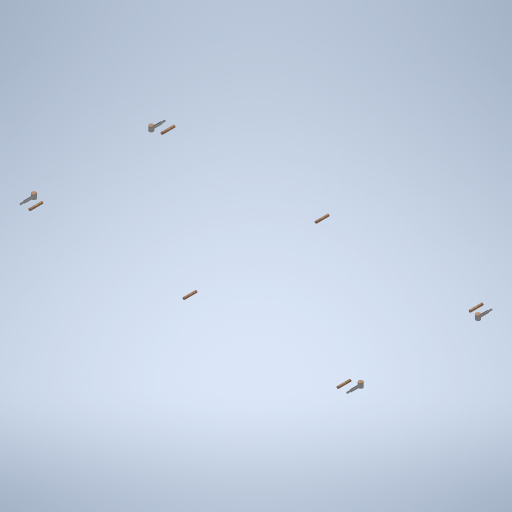
# Autodesk Inventor part: Minifixes pull Side Boards-04
Saved by Autodesk Inventor 2024.3 (Build 283343000, 343)
## iProperties
RuleStatus: InUse
Created: 2014-05-08
Part Number: Minifixes pull Side Boards-04
Material: Generic
Document SubType Name: Modeling
Designer: SauliusD
Density: 1 g/cm^3
Appearance: Default
AfterDocNew0: Fire Form
Author: SauliusD
Autodesk Inventor part; units mm, degrees
sketch "Sketch2" plane through (0, 0, 0) normal (0, 0, 1) x (1, 0, 0)
  line L0 (-178.2411, -363.1253) -> (-1324.2411, -363.1253)
  line L1 (-1324.2411, -363.1253) -> (-1324.2411, 106.8747)
  line L2 (-1324.2411, 106.8747) -> (-178.2411, 106.8747)
  line L3 (-178.2411, 106.8747) -> (-178.2411, -363.1253)
  point P0 (-751.2411, 106.8747)
  point P1 (-1324.2411, -128.1253)
  constraints: 8 end point, 2 midpoint, 2 parallel, 1 horizontal, 1 perpendicular
ref_plane "Work Plane1" through (0, 0, -9) normal (0, 0, 1) x (1, 0, 0)
sketch "Sketch3" plane through (0, 0, -9) normal (0, 0, 1) x (1, 0, 0)
  line L0 (-178.2411, 106.8747) -> (-178.2411, -363.1253) construction
  line L1 (-1324.2411, 106.8747) -> (-178.2411, 106.8747) construction
  line L2 (-1324.2411, -363.1253) -> (-1324.2411, 106.8747) construction
  line L3 (-1311.2411, 106.8747) -> (-1307.2411, 106.8747)
  line L4 (-1307.2411, 106.8747) -> (-1307.2411, 72.8747)
  line L5 (-1307.2411, 72.8747) -> (-1311.2411, 72.8747)
  line L6 (-1311.2411, 72.8747) -> (-1311.2411, 106.8747)
  line L7 (-1311.2411, 106.8747) -> (-1308.7411, 106.8747)
  line L8 (-1308.7411, 106.8747) -> (-1308.7411, 119.8747)
  line L9 (-1308.7411, 119.8747) -> (-1311.2411, 119.8747)
  line L10 (-1311.2411, 119.8747) -> (-1311.2411, 106.8747)
  line L11 (-751.2411, 106.8747) -> (-751.2411, 132.7708) construction
  line L12 (-191.2411, 72.8747) -> (-191.2411, 106.8747)
  point P0 (0, 0)
  dimension "d5" = 8
  dimension "d7" = 5
  dimension "d8" = 13
  dimension "Dist_Between_Planes" = 1146
  dimension "Distance_between_Axis" = 1120
  constraints: 20 end point, 5 parallel, 2 horizontal, 2 perpendicular, 2 symmetric about line, 1 collinear, 1 midpoint, 1 vertical alignment
  measures "d5" diameter of L4 L6
  measures "d7" diameter of L8 L10
  measures "d8" distance of L7.end L8.end
  measures "Dist_Between_Planes" distance of L1.start L0.start
  measures "Distance_between_Axis" distance between parallel lines of L6 L12
revolve "Minifix Revolve" add sketch "Sketch3" angle 360 about axis through (-1311.2411, 119.8747, -9) along (0, -1, 0)
sketch "Sketch4" plane through (0, 0, -9) normal (0, 0, 1) x (1, 0, 0)
  line L0 (-1315.2411, 72.8747) -> (-1307.2411, 72.8747) construction
  circle A0 centre (-1311.2411, 72.8747) radius 7.5
  point P0 (0, 0)
  dimension "d10" = 15
  constraints: 1 centre point, 1 midpoint
  measures "d10" diameter of A0
extrude "Minifix Extrude" add sketch "Sketch4" along normal up to surface (9 mm away)
extrude "Minifix extrude 2" add sketch "Sketch4" against normal blind 6
ref_plane "Work Plane2" through (-751.2411, 106.8747, 0) normal (1, 0, 0) x (0, 1, 0)
ref_plane "Work Plane3" through (-1324.2411, -128.1253, 0) normal (0, 1, 0) x (-1, 0, 0)
sketch "Sketch5" plane through (0, 0, -9) normal (0, 0, 1) x (1, 0, 0)
  line L0 (-1311.2411, 216.4747) -> (-1311.2411, -459.7253) construction
  line L1 (-1279.2411, 119.8747) -> (-1279.2411, 76.8747)
  line L2 (-1279.2411, 119.8747) -> (-1275.2411, 119.8747)
  line L3 (-1275.2411, 119.8747) -> (-1275.2411, 76.8747)
  line L4 (-1275.2411, 76.8747) -> (-1279.2411, 76.8747)
  line L5 (-1313.7411, 119.8747) -> (-1308.7411, 119.8747) construction
  line L6 (-1315.2411, 106.8747) -> (-1307.2411, 106.8747) construction
  point P0 (0, 0)
  dimension "Dowel_D" = 8
  dimension "Dowel_Drill_Depth" = 30
  dimension "d17" = 32
  constraints: 8 end point, 2 parallel, 2 perpendicular, 1 collinear
  measures "Dowel_D" diameter of L3 L1
  measures "Dowel_Drill_Depth" distance between parallel lines of L4 L6
  measures "d17" distance from line of L1.start L0
revolve "Dowel Revolve" add sketch "Sketch5" angle 360 about axis through (-1279.2411, 119.8747, -9) along (0, -1, 0) separate body
mirror "Mirror1" about plane through (-751.2411, 106.8747, 0) normal (1, 0, 0) of "Minifix Extrude", "Minifix Revolve", "Dowel Revolve", "Minifix extrude 2" bodies 1
sketch "Sketch6" plane through (0, 0, -9) normal (0, 0, 1) x (1, 0, 0)
  point P0 (0, 0)
sketch "Sketch7" plane through (0, 0, -9) normal (0, 0, 1) x (1, 0, 0)
  line L0 (-751.2411, 216.4747) -> (-751.2411, -459.7253) construction
  line L1 (-751.2411, 119.8747) -> (-747.2411, 119.8747)
  line L2 (-747.2411, 119.8747) -> (-747.2411, 76.8747)
  line L3 (-747.2411, 76.8747) -> (-751.2411, 76.8747)
  line L4 (-751.2411, 76.8747) -> (-751.2411, 119.8747)
  line L5 (-1313.7411, 119.8747) -> (-1308.7411, 119.8747) construction
  line L6 (-1315.2411, 106.8747) -> (-1307.2411, 106.8747) construction
  line L7 (-1283.2411, 76.8747) -> (-1275.2411, 76.8747) projected
  line L8 (-1283.2411, 119.8747) -> (-1275.2411, 119.8747) projected
  point P0 (0, 0)
  point P1 (-751.2411, -459.7253)
  dimension "d46" = 8
  constraints: 8 end point, 2 collinear, 2 parallel, 1 horizontal, 1 perpendicular, 1 vertical, 1 other
  measures "d46" diameter of L2 L4
revolve "Center Dowel Revolve" add sketch "Sketch7" angle 360 about axis through (-751.2411, 106.8747, -9) along (0, -1, 0) separate body
ref_plane "Work Plane4" through (-178.2411, 106.8747, 0) normal (0, 1, 0) x (-1, 0, 0)
mirror "Mirror2" about plane through (-1324.2411, -128.1253, 0) normal (0, 1, 0) of "Minifix Extrude", "Minifix Revolve", "Dowel Revolve", "Minifix extrude 2", "Mirror1" bodies 1
mirror "Mirror Center" about plane through (-1324.2411, -128.1253, 0) normal (0, 1, 0) of "Center Dowel Revolve" bodies 3
sketch "Sketch9" plane through (-1311.2411, 72.8747, 0) normal (0, 0, 1) x (1, 0, 0)
  circle A0 centre (0, 0) radius 7.5 projected
  point P0 (1311.2411, -72.8747)
extrude "Side Cover Cap Extrusion" add sketch "Sketch9" along normal blind 2 separate body
fillet "Side Cover Cap Fillet" radius 1.6 1 edges at (-1318.7411, 72.8747, 2)
mirror "Mirror3" about plane through (-751.2411, 106.8747, 0) normal (1, 0, 0) of "Side Cover Cap Extrusion", "Side Cover Cap Fillet" bodies 4
mirror "Mirror4" about plane through (-1324.2411, -128.1253, 0) normal (0, 1, 0) of "Side Cover Cap Extrusion", "Side Cover Cap Fillet", "Mirror3" bodies 4
equation "\"d46\" = Dowel_D"
equation "\"Step\" = 32"
